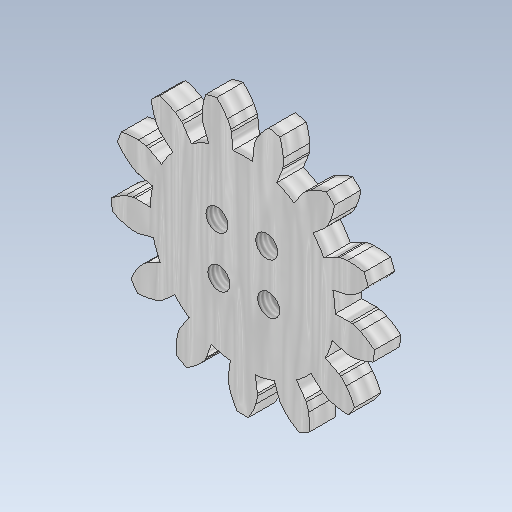
# Autodesk Inventor part: ｍ2歯数13ギアd10同軸ネジ切甲
Saved by Autodesk Inventor 2020.2 (Build 242310000, 310)
## iProperties
Created: 2020-02-11
Part Number: ｍ2歯数13ギアd10同軸ネジ切甲
Material: アルミニウム 7075
Document SubType Name: Modeling
Designer: aoyam
Density: 2.81 g/cm^3
Appearance: サテン - ブラシ仕上げ 重厚
Author: aoyam
Autodesk Inventor part; units mm, degrees
ref_plane "YZ Plane" through (0, 0, 0) normal (1, 0, 0) x (0, 1, 0)
ref_plane "XZ Plane" through (0, 0, 0) normal (0, 1, 0) x (-1, 0, 0)
ref_plane "XY Plane" through (0, 0, 0) normal (0, 0, 1) x (1, 0, 0)
sketch "スケッチ1" plane through (0, 0, 0) normal (0, 0, 1) x (1, 0, 0)
  arc A0 (149.8566, 117.4069) -> (149.7916, 117.1475) centre (151.2088, 116.9303) ccw
  arc A1 (150.243, 118.2214) -> (149.8566, 117.4069) centre (153.6231, 116.1188) ccw
  arc A2 (151.4709, 119.7028) -> (150.243, 118.2214) centre (156.2171, 114.5193) ccw
  arc A3 (147.2084, 117.1475) -> (147.1434, 117.4069) centre (145.7912, 116.9303) ccw
  arc A4 (147.1434, 117.4069) -> (146.757, 118.2214) centre (143.3769, 116.1188) ccw
  arc A5 (146.757, 118.2214) -> (145.5291, 119.7028) centre (140.7829, 114.5193) ccw
  arc A6 (149.6101, 115.4411) -> (147.3899, 115.4411) centre (148.5, 105) ccw
  arc A7 (145.5291, 119.7028) -> (144.2978, 119.3994) centre (148.5, 105) ccw
  line L0 (149.6101, 115.4411) -> (149.7916, 117.1475)
  line L1 (147.3899, 115.4411) -> (147.2084, 117.1475)
  line L2 (131.5, 105) -> (165.5, 105)
  line L3 (148.5, 88) -> (148.5, 122)
  arc A8 (143.9354, 116.6162) -> (143.9984, 116.3563) centre (145.3542, 116.8225) ccw
  line L4 (144.6307, 114.7611) -> (143.9984, 116.3563)
  arc A9 (143.8991, 117.517) -> (143.9354, 116.6162) centre (147.8691, 117.226) ccw
  arc A10 (144.2978, 119.3994) -> (143.8991, 117.517) centre (150.9093, 117.0153) ccw
  arc A11 (144.6307, 114.7611) -> (142.6648, 113.7293) centre (148.5, 105) ccw
  line L5 (142.6648, 113.7293) -> (141.7111, 115.1559)
  arc A12 (141.7111, 115.1559) -> (141.5331, 115.3553) centre (140.5572, 114.3049) ccw
  arc A13 (141.5331, 115.3553) -> (140.8123, 115.897) centre (138.7966, 112.4644) ccw
  arc A14 (140.8123, 115.897) -> (139.0366, 116.6381) centre (137.2429, 109.8426) ccw
  arc A15 (139.0366, 116.6381) -> (138.0875, 115.7972) centre (148.5, 105) ccw
  arc A16 (139.0599, 113.1643) -> (139.2365, 112.9635) centre (140.2203, 114.0064) ccw
  line L6 (140.5377, 111.8449) -> (139.2365, 112.9635)
  arc A17 (138.6091, 113.9451) -> (139.0599, 113.1643) centre (142.2596, 115.5324) ccw
  arc A18 (138.0875, 115.7972) -> (138.6091, 113.9451) centre (145.0496, 116.7587) ccw
  arc A19 (140.5377, 111.8449) -> (139.2765, 110.0176) centre (148.5, 105) ccw
  line L7 (139.2765, 110.0176) -> (137.7691, 110.8376)
  arc A20 (137.7691, 110.8376) -> (137.5187, 110.9315) centre (137.1428, 109.5479) ccw
  arc A21 (137.5187, 110.9315) -> (136.6288, 111.0762) centre (136.4392, 107.1) ccw
  arc A22 (136.6288, 111.0762) -> (134.7121, 110.9072) centre (136.2819, 104.0565) ccw
  arc A23 (134.7121, 110.9072) -> (134.2625, 109.7215) centre (148.5, 105) ccw
  arc A24 (136.3471, 107.8422) -> (136.5967, 107.7464) centre (136.9832, 109.127) ccw
  line L8 (138.2688, 107.3606) -> (136.5967, 107.7464)
  arc A25 (135.585, 108.324) -> (136.3471, 107.8422) centre (138.0798, 111.426) ccw
  arc A26 (134.2625, 109.7215) -> (135.585, 108.324) centre (139.9803, 113.8083) ccw
  arc A27 (138.2688, 107.3606) -> (138.0012, 105.1565) centre (148.5, 105) ccw
  line L9 (138.0012, 105.1565) -> (136.2854, 105.1821)
  arc A28 (136.2854, 105.1821) -> (136.0201, 105.1488) centre (136.3302, 103.749) ccw
  arc A29 (136.0201, 105.1488) -> (135.1649, 104.8633) centre (136.8447, 101.2545) ccw
  arc A30 (135.1649, 104.8633) -> (133.5462, 103.823) centre (138.1199, 98.4866) ccw
  arc A31 (133.5462, 103.823) -> (133.6991, 102.5641) centre (148.5, 105) ccw
  arc A32 (136.4183, 101.8689) -> (136.6839, 101.9001) centre (136.3845, 103.3022) ccw
  line L10 (138.3437, 102.3355) -> (136.6839, 101.9001)
  arc A33 (135.5196, 101.9414) -> (136.4183, 101.8689) centre (136.2871, 105.8474) ccw
  arc A34 (133.6991, 102.5641) -> (135.5196, 101.9414) centre (136.8627, 108.84) ccw
  arc A35 (138.3437, 102.3355) -> (139.131, 100.2595) centre (148.5, 105) ccw
  line L11 (139.131, 100.2595) -> (137.5999, 99.4848)
  arc A36 (137.5999, 99.4848) -> (137.3804, 99.3321) centre (138.3055, 98.2367) ccw
  arc A37 (137.3804, 99.3321) -> (136.7558, 98.6818) centre (139.9204, 96.2671) ccw
  arc A38 (136.7558, 98.6818) -> (135.8061, 97.0085) centre (142.3358, 94.4087) ccw
  arc A39 (135.8061, 97.0085) -> (136.5265, 95.9648) centre (148.5, 105) ccw
  arc A40 (139.2573, 96.6129) -> (139.4779, 96.7639) centre (138.5612, 97.8663) ccw
  line L12 (140.7453, 97.9209) -> (139.4779, 96.7639)
  arc A41 (138.4279, 96.2594) -> (139.2573, 96.6129) centre (137.2922, 100.0747) ccw
  arc A42 (136.5265, 95.9648) -> (138.4279, 96.2594) centre (136.4111, 102.9921) ccw
  arc A43 (140.7453, 97.9209) -> (142.4072, 96.4485) centre (148.5, 105) ccw
  line L13 (142.4072, 96.4485) -> (141.4115, 95.051)
  arc A44 (141.4115, 95.051) -> (141.2881, 94.8138) centre (142.6163, 94.2738) ccw
  arc A45 (141.2881, 94.8138) -> (141.0372, 93.9478) centre (144.9616, 93.2802) ccw
  arc A46 (141.0372, 93.9478) -> (140.974, 92.0247) centre (147.9639, 92.7573) ccw
  arc A47 (140.974, 92.0247) -> (142.0968, 91.4354) centre (148.5, 105) ccw
  arc A48 (144.2137, 93.2783) -> (144.3389, 93.5145) centre (143.0149, 94.0647) ccw
  line L14 (144.9234, 95.1279) -> (144.3389, 93.5145)
  arc A49 (143.6435, 92.5799) -> (144.2137, 93.2783) centre (140.8649, 95.4303) ccw
  arc A50 (142.0968, 91.4354) -> (143.6435, 92.5799) centre (138.729, 97.6041) ccw
  arc A51 (144.9234, 95.1279) -> (147.0792, 94.5966) centre (148.5, 105) ccw
  line L15 (147.0792, 94.5966) -> (146.8469, 92.8964)
  arc A52 (146.8469, 92.8964) -> (146.848, 92.629) centre (148.2749, 92.7682) ccw
  arc A53 (146.848, 92.629) -> (147.0283, 91.7456) centre (150.8133, 92.9783) ccw
  arc A54 (147.0283, 91.7456) -> (147.8659, 90.0134) centre (153.7148, 93.9104) ccw
  arc A55 (147.8659, 90.0134) -> (149.1341, 90.0134) centre (148.5, 105) ccw
  arc A56 (150.152, 92.629) -> (150.1531, 92.8964) centre (148.7251, 92.7682) ccw
  line L16 (149.9208, 94.5966) -> (150.1531, 92.8964)
  arc A57 (149.9717, 91.7456) -> (150.152, 92.629) centre (146.1867, 92.9783) ccw
  arc A58 (149.1341, 90.0134) -> (149.9717, 91.7456) centre (143.2852, 93.9104) ccw
  arc A59 (149.9208, 94.5966) -> (152.0766, 95.1279) centre (148.5, 105) ccw
  line L17 (152.0766, 95.1279) -> (152.6611, 93.5145)
  arc A60 (152.6611, 93.5145) -> (152.7863, 93.2783) centre (153.9851, 94.0647) ccw
  arc A61 (152.7863, 93.2783) -> (153.3565, 92.5799) centre (156.1351, 95.4303) ccw
  arc A62 (153.3565, 92.5799) -> (154.9032, 91.4354) centre (158.271, 97.6041) ccw
  arc A63 (154.9032, 91.4354) -> (156.026, 92.0247) centre (148.5, 105) ccw
  arc A64 (155.7119, 94.8138) -> (155.5885, 95.051) centre (154.3837, 94.2738) ccw
  line L18 (154.5928, 96.4485) -> (155.5885, 95.051)
  arc A65 (155.9628, 93.9478) -> (155.7119, 94.8138) centre (152.0384, 93.2802) ccw
  arc A66 (156.026, 92.0247) -> (155.9628, 93.9478) centre (149.0361, 92.7573) ccw
  arc A67 (154.5928, 96.4485) -> (156.2547, 97.9209) centre (148.5, 105) ccw
  line L19 (156.2547, 97.9209) -> (157.5221, 96.7639)
  arc A68 (157.5221, 96.7639) -> (157.7427, 96.6129) centre (158.4388, 97.8663) ccw
  arc A69 (157.7427, 96.6129) -> (158.5721, 96.2594) centre (159.7078, 100.0747) ccw
  arc A70 (158.5721, 96.2594) -> (160.4735, 95.9648) centre (160.5889, 102.9921) ccw
  arc A71 (160.4735, 95.9648) -> (161.1939, 97.0085) centre (148.5, 105) ccw
  arc A72 (159.6196, 99.3321) -> (159.4001, 99.4848) centre (158.6945, 98.2367) ccw
  line L20 (157.869, 100.2595) -> (159.4001, 99.4848)
  arc A73 (160.2442, 98.6818) -> (159.6196, 99.3321) centre (157.0796, 96.2671) ccw
  arc A74 (161.1939, 97.0085) -> (160.2442, 98.6818) centre (154.6642, 94.4087) ccw
  arc A75 (157.869, 100.2595) -> (158.6563, 102.3355) centre (148.5, 105) ccw
  line L21 (158.6563, 102.3355) -> (160.3161, 101.9001)
  arc A76 (160.3161, 101.9001) -> (160.5817, 101.8689) centre (160.6155, 103.3022) ccw
  arc A77 (160.5817, 101.8689) -> (161.4804, 101.9414) centre (160.7129, 105.8474) ccw
  arc A78 (161.4804, 101.9414) -> (163.3009, 102.5641) centre (160.1373, 108.84) ccw
  arc A79 (163.3009, 102.5641) -> (163.4538, 103.823) centre (148.5, 105) ccw
  arc A80 (160.9799, 105.1488) -> (160.7146, 105.1821) centre (160.6698, 103.749) ccw
  line L22 (158.9988, 105.1565) -> (160.7146, 105.1821)
  arc A81 (161.8351, 104.8633) -> (160.9799, 105.1488) centre (160.1553, 101.2545) ccw
  arc A82 (163.4538, 103.823) -> (161.8351, 104.8633) centre (158.8801, 98.4866) ccw
  arc A83 (158.9988, 105.1565) -> (158.7312, 107.3606) centre (148.5, 105) ccw
  line L23 (158.7312, 107.3606) -> (160.4033, 107.7464)
  arc A84 (160.4033, 107.7464) -> (160.6529, 107.8422) centre (160.0168, 109.127) ccw
  arc A85 (160.6529, 107.8422) -> (161.415, 108.324) centre (158.9202, 111.426) ccw
  arc A86 (161.415, 108.324) -> (162.7375, 109.7215) centre (157.0197, 113.8083) ccw
  arc A87 (162.7375, 109.7215) -> (162.2879, 110.9072) centre (148.5, 105) ccw
  arc A88 (159.4813, 110.9315) -> (159.2309, 110.8376) centre (159.8572, 109.5479) ccw
  line L24 (157.7235, 110.0176) -> (159.2309, 110.8376)
  arc A89 (160.3712, 111.0762) -> (159.4813, 110.9315) centre (160.5608, 107.1) ccw
  arc A90 (162.2879, 110.9072) -> (160.3712, 111.0762) centre (160.7181, 104.0565) ccw
  arc A91 (157.7235, 110.0176) -> (156.4623, 111.8449) centre (148.5, 105) ccw
  line L25 (156.4623, 111.8449) -> (157.7635, 112.9635)
  arc A92 (157.7635, 112.9635) -> (157.9401, 113.1643) centre (156.7797, 114.0064) ccw
  arc A93 (157.9401, 113.1643) -> (158.3909, 113.9451) centre (154.7404, 115.5324) ccw
  arc A94 (158.3909, 113.9451) -> (158.9125, 115.7972) centre (151.9504, 116.7587) ccw
  arc A95 (158.9125, 115.7972) -> (157.9634, 116.6381) centre (148.5, 105) ccw
  arc A96 (155.4669, 115.3553) -> (155.2889, 115.1559) centre (156.4428, 114.3049) ccw
  line L26 (154.3352, 113.7293) -> (155.2889, 115.1559)
  arc A97 (156.1877, 115.897) -> (155.4669, 115.3553) centre (158.2034, 112.4644) ccw
  arc A98 (157.9634, 116.6381) -> (156.1877, 115.897) centre (159.7571, 109.8426) ccw
  arc A99 (154.3352, 113.7293) -> (152.3693, 114.7611) centre (148.5, 105) ccw
  line L27 (152.3693, 114.7611) -> (153.0016, 116.3563)
  arc A100 (153.0016, 116.3563) -> (153.0646, 116.6162) centre (151.6458, 116.8225) ccw
  arc A101 (153.0646, 116.6162) -> (153.1009, 117.517) centre (149.1309, 117.226) ccw
  arc A102 (153.1009, 117.517) -> (152.7022, 119.3994) centre (146.0907, 117.0153) ccw
  arc A103 (152.7022, 119.3994) -> (151.4709, 119.7028) centre (148.5, 105) ccw
  circle A104 centre (148.5, 105) radius 10.5
  circle A105 centre (148.5, 105) radius 7.75 construction
  circle A106 centre (145.5628, 107.7153) radius 1.25
  circle A107 centre (145.7847, 102.0628) radius 1.25
  circle A108 centre (151.4372, 102.2847) radius 1.25
  circle A109 centre (151.2153, 107.9372) radius 1.25
  line L28 (142.8007, 109.2819) -> (145.5384, 110.8906)
  line L29 (145.5384, 110.8906) -> (148.3005, 109.324)
  line L30 (148.3005, 109.324) -> (148.3249, 106.1487)
  line L31 (148.3249, 106.1487) -> (145.5871, 104.5399)
  line L32 (145.5871, 104.5399) -> (142.825, 106.1065)
  line L33 (142.825, 106.1065) -> (142.8007, 109.2819)
  circle A110 centre (145.5628, 107.7153) radius 3.1754
  circle A111 centre (151.2153, 107.9372) radius 2.75
  point P0 (0, 0)
  point P1 (140.5997, 120.0528)
  point P2 (134.5093, 114.6571)
  point P3 (131.6239, 107.0491)
  point P4 (132.6047, 98.9717)
  point P5 (137.2269, 92.2753)
  point P6 (144.4316, 88.494)
  point P7 (152.5684, 88.494)
  point P8 (159.7731, 92.2753)
  point P9 (164.3953, 98.9717)
  point P10 (165.3761, 107.0491)
  point P11 (162.4907, 114.6571)
  point P12 (156.4003, 120.0528)
  point P13 (149.1341, 90.0134)
  point P14 (149.9717, 91.7456)
  point P15 (150.152, 92.629)
  point P16 (149.9208, 94.5966)
  point P17 (152.7863, 93.2783)
  point P18 (153.3565, 92.5799)
  point P19 (154.9032, 91.4354)
  point P20 (156.026, 92.0247)
  point P21 (155.9628, 93.9478)
  point P22 (154.5928, 96.4485)
  point P23 (157.5221, 96.7639)
  point P24 (157.7427, 96.6129)
  point P25 (158.5721, 96.2594)
  point P26 (160.4735, 95.9648)
  point P27 (161.1939, 97.0085)
  point P28 (160.2442, 98.6818)
  point P29 (160.3161, 101.9001)
  point P30 (160.5817, 101.8689)
  point P31 (161.4804, 101.9414)
  point P32 (161.8351, 104.8633)
  point P33 (160.6529, 107.8422)
  point P34 (162.7375, 109.7215)
  point P35 (162.2879, 110.9072)
  point P36 (160.3712, 111.0762)
  point P37 (159.4813, 110.9315)
  point P38 (157.7235, 110.0176)
  point P39 (157.7635, 112.9635)
  point P40 (157.9401, 113.1643)
  point P41 (158.3909, 113.9451)
  point P42 (158.9125, 115.7972)
  point P43 (154.3352, 113.7293)
  point P44 (153.0016, 116.3563)
  point P45 (152.7022, 119.3994)
  point P46 (151.4709, 119.7028)
  point P47 (150.243, 118.2214)
  point P48 (149.8566, 117.4069)
  point P49 (147.3899, 115.4411)
  point P50 (146.757, 118.2214)
  point P51 (144.2978, 119.3994)
  point P52 (143.8991, 117.517)
  point P53 (144.6307, 114.7611)
  point P54 (140.8123, 115.897)
  point P55 (139.0366, 116.6381)
  point P56 (138.0875, 115.7972)
  point P57 (138.6091, 113.9451)
  point P58 (139.0599, 113.1643)
  point P59 (140.5377, 111.8449)
  point P60 (137.7691, 110.8376)
  point P61 (137.5187, 110.9315)
  point P62 (136.6288, 111.0762)
  point P63 (134.7121, 110.9072)
  point P64 (134.2625, 109.7215)
  point P65 (135.585, 108.324)
  point P66 (138.2688, 107.3606)
  point P67 (133.5462, 103.823)
  point P68 (133.6991, 102.5641)
  point P69 (135.5196, 101.9414)
  point P70 (136.4183, 101.8689)
  point P71 (138.3437, 102.3355)
  point P72 (137.5999, 99.4848)
  point P73 (137.3804, 99.3321)
  point P74 (142.0968, 91.4354)
  point P75 (144.2137, 93.2783)
  point P76 (147.8659, 90.0134)
  dimension "d25" = 6.3509
  dimension "d2" = 360
  dimension "d16" = 2.5
  dimension "d17" = 4
  dimension "d20" = 360
  dimension "d24" = 5.5
  dimension "d26" = 5.5
  constraints: 208 point on circle, 111 centre point, 68 end point, 6 coincident, 1 concentric, 1 midpoint, 532 other
  measures "d16" diameter of A106
  measures "d17" distance of A6.centre A106.centre
  measures "d24" distance between parallel lines of L32 L29
  measures "d26" diameter of A111
extrude "押し出し1" add sketch "スケッチ1" along normal blind 3
sketch "スケッチ2" plane through (0, 0, 0) normal (0, 0, -1) x (-1, 0, 0)
  point P0 (0, 0)
sketch "スケッチ3" plane through (0, 0, 3) normal (0, 0, 1) x (1, 0, 0)
  arc A0 (138.4279, 96.2594) -> (139.2573, 96.6129) centre (137.2922, 100.0747) ccw projected
  arc A1 (139.2573, 96.6129) -> (139.4779, 96.7639) centre (138.5612, 97.8663) ccw projected
  line L0 (139.4779, 96.7639) -> (140.7453, 97.9209) projected
  arc A2 (140.7453, 97.9209) -> (142.4072, 96.4485) centre (148.5, 105) ccw projected
  line L1 (142.4072, 96.4485) -> (141.4115, 95.051) projected
  arc A3 (141.4115, 95.051) -> (141.2881, 94.8138) centre (142.6163, 94.2738) ccw projected
  arc A4 (141.2881, 94.8138) -> (141.0372, 93.9478) centre (144.9616, 93.2802) ccw projected
  arc A5 (141.0372, 93.9478) -> (140.974, 92.0247) centre (147.9639, 92.7573) ccw projected
  arc A6 (140.974, 92.0247) -> (142.0968, 91.4354) centre (148.5, 105) ccw projected
  arc A7 (142.0968, 91.4354) -> (143.6435, 92.5799) centre (138.729, 97.6041) ccw projected
  arc A8 (143.6435, 92.5799) -> (144.2137, 93.2783) centre (140.8649, 95.4303) ccw projected
  arc A9 (144.2137, 93.2783) -> (144.3389, 93.5145) centre (143.0149, 94.0647) ccw projected
  line L2 (144.3389, 93.5145) -> (144.9234, 95.1279) projected
  arc A10 (144.9234, 95.1279) -> (147.0792, 94.5966) centre (148.5, 105) ccw projected
  line L3 (147.0792, 94.5966) -> (146.8469, 92.8964) projected
  arc A11 (146.8469, 92.8964) -> (146.848, 92.629) centre (148.2749, 92.7682) ccw projected
  arc A12 (146.848, 92.629) -> (147.0283, 91.7456) centre (150.8133, 92.9783) ccw projected
  arc A13 (147.0283, 91.7456) -> (147.8659, 90.0134) centre (153.7148, 93.9104) ccw projected
  arc A14 (147.8659, 90.0134) -> (149.1341, 90.0134) centre (148.5, 105) ccw projected
  arc A15 (149.1341, 90.0134) -> (149.9717, 91.7456) centre (143.2852, 93.9104) ccw projected
  arc A16 (149.9717, 91.7456) -> (150.152, 92.629) centre (146.1867, 92.9783) ccw projected
  arc A17 (150.152, 92.629) -> (150.1531, 92.8964) centre (148.7251, 92.7682) ccw projected
  line L4 (150.1531, 92.8964) -> (149.9208, 94.5966) projected
  arc A18 (149.9208, 94.5966) -> (152.0766, 95.1279) centre (148.5, 105) ccw projected
  line L5 (152.0766, 95.1279) -> (152.6611, 93.5145) projected
  arc A19 (152.6611, 93.5145) -> (152.7863, 93.2783) centre (153.9851, 94.0647) ccw projected
  arc A20 (152.7863, 93.2783) -> (153.3565, 92.5799) centre (156.1351, 95.4303) ccw projected
  arc A21 (153.3565, 92.5799) -> (154.9032, 91.4354) centre (158.271, 97.6041) ccw projected
  arc A22 (154.9032, 91.4354) -> (156.026, 92.0247) centre (148.5, 105) ccw projected
  arc A23 (156.026, 92.0247) -> (155.9628, 93.9478) centre (149.0361, 92.7573) ccw projected
  arc A24 (155.9628, 93.9478) -> (155.7119, 94.8138) centre (152.0384, 93.2802) ccw projected
  arc A25 (155.7119, 94.8138) -> (155.5885, 95.051) centre (154.3837, 94.2738) ccw projected
  line L6 (155.5885, 95.051) -> (154.5928, 96.4485) projected
  arc A26 (154.5928, 96.4485) -> (156.2547, 97.9209) centre (148.5, 105) ccw projected
  line L7 (156.2547, 97.9209) -> (157.5221, 96.7639) projected
  arc A27 (157.5221, 96.7639) -> (157.7427, 96.6129) centre (158.4388, 97.8663) ccw projected
  arc A28 (157.7427, 96.6129) -> (158.5721, 96.2594) centre (159.7078, 100.0747) ccw projected
  arc A29 (158.5721, 96.2594) -> (160.4735, 95.9648) centre (160.5889, 102.9921) ccw projected
  arc A30 (160.4735, 95.9648) -> (161.1939, 97.0085) centre (148.5, 105) ccw projected
  arc A31 (161.1939, 97.0085) -> (160.2442, 98.6818) centre (154.6642, 94.4087) ccw projected
  arc A32 (160.2442, 98.6818) -> (159.6196, 99.3321) centre (157.0796, 96.2671) ccw projected
  arc A33 (159.6196, 99.3321) -> (159.4001, 99.4848) centre (158.6945, 98.2367) ccw projected
  line L8 (159.4001, 99.4848) -> (157.869, 100.2595) projected
  arc A34 (157.869, 100.2595) -> (158.6563, 102.3355) centre (148.5, 105) ccw projected
  line L9 (158.6563, 102.3355) -> (160.3161, 101.9001) projected
  arc A35 (160.3161, 101.9001) -> (160.5817, 101.8689) centre (160.6155, 103.3022) ccw projected
  arc A36 (160.5817, 101.8689) -> (161.4804, 101.9414) centre (160.7129, 105.8474) ccw projected
  arc A37 (161.4804, 101.9414) -> (163.3009, 102.5641) centre (160.1373, 108.84) ccw projected
  arc A38 (163.3009, 102.5641) -> (163.4538, 103.823) centre (148.5, 105) ccw projected
  arc A39 (163.4538, 103.823) -> (161.8351, 104.8633) centre (158.8801, 98.4866) ccw projected
  arc A40 (161.8351, 104.8633) -> (160.9799, 105.1488) centre (160.1553, 101.2545) ccw projected
  arc A41 (160.9799, 105.1488) -> (160.7146, 105.1821) centre (160.6698, 103.749) ccw projected
  line L10 (160.7146, 105.1821) -> (158.9988, 105.1565) projected
  arc A42 (158.9988, 105.1565) -> (158.7312, 107.3606) centre (148.5, 105) ccw projected
  line L11 (158.7312, 107.3606) -> (160.4033, 107.7464) projected
  arc A43 (160.4033, 107.7464) -> (160.6529, 107.8422) centre (160.0168, 109.127) ccw projected
  arc A44 (160.6529, 107.8422) -> (161.415, 108.324) centre (158.9202, 111.426) ccw projected
  arc A45 (161.415, 108.324) -> (162.7375, 109.7215) centre (157.0197, 113.8083) ccw projected
  arc A46 (162.7375, 109.7215) -> (162.2879, 110.9072) centre (148.5, 105) ccw projected
  arc A47 (162.2879, 110.9072) -> (160.3712, 111.0762) centre (160.7181, 104.0565) ccw projected
  arc A48 (160.3712, 111.0762) -> (159.4813, 110.9315) centre (160.5608, 107.1) ccw projected
  arc A49 (159.4813, 110.9315) -> (159.2309, 110.8376) centre (159.8572, 109.5479) ccw projected
  line L12 (159.2309, 110.8376) -> (157.7235, 110.0176) projected
  arc A50 (157.7235, 110.0176) -> (156.4623, 111.8449) centre (148.5, 105) ccw projected
  line L13 (156.4623, 111.8449) -> (157.7635, 112.9635) projected
  arc A51 (157.7635, 112.9635) -> (157.9401, 113.1643) centre (156.7797, 114.0064) ccw projected
  arc A52 (157.9401, 113.1643) -> (158.3909, 113.9451) centre (154.7404, 115.5324) ccw projected
  arc A53 (158.3909, 113.9451) -> (158.9125, 115.7972) centre (151.9504, 116.7587) ccw projected
  arc A54 (158.9125, 115.7972) -> (157.9634, 116.6381) centre (148.5, 105) ccw projected
  arc A55 (157.9634, 116.6381) -> (156.1877, 115.897) centre (159.7571, 109.8426) ccw projected
  arc A56 (156.1877, 115.897) -> (155.4669, 115.3553) centre (158.2034, 112.4644) ccw projected
  arc A57 (155.4669, 115.3553) -> (155.2889, 115.1559) centre (156.4428, 114.3049) ccw projected
  line L14 (155.2889, 115.1559) -> (154.3352, 113.7293) projected
  arc A58 (154.3352, 113.7293) -> (152.3693, 114.7611) centre (148.5, 105) ccw projected
  line L15 (152.3693, 114.7611) -> (153.0016, 116.3563) projected
  arc A59 (153.0016, 116.3563) -> (153.0646, 116.6162) centre (151.6458, 116.8225) ccw projected
  arc A60 (153.0646, 116.6162) -> (153.1009, 117.517) centre (149.1309, 117.226) ccw projected
  arc A61 (153.1009, 117.517) -> (152.7022, 119.3994) centre (146.0907, 117.0153) ccw projected
  arc A62 (152.7022, 119.3994) -> (151.4709, 119.7028) centre (148.5, 105) ccw projected
  arc A63 (151.4709, 119.7028) -> (150.243, 118.2214) centre (156.2171, 114.5193) ccw projected
  arc A64 (150.243, 118.2214) -> (149.8566, 117.4069) centre (153.6231, 116.1188) ccw projected
  arc A65 (149.8566, 117.4069) -> (149.7916, 117.1475) centre (151.2088, 116.9303) ccw projected
  line L16 (149.7916, 117.1475) -> (149.6101, 115.4411) projected
  arc A66 (149.6101, 115.4411) -> (147.3899, 115.4411) centre (148.5, 105) ccw projected
  line L17 (147.3899, 115.4411) -> (147.2084, 117.1475) projected
  arc A67 (147.2084, 117.1475) -> (147.1434, 117.4069) centre (145.7912, 116.9303) ccw projected
  arc A68 (147.1434, 117.4069) -> (146.757, 118.2214) centre (143.3769, 116.1188) ccw projected
  arc A69 (146.757, 118.2214) -> (145.5291, 119.7028) centre (140.7829, 114.5193) ccw projected
  arc A70 (145.5291, 119.7028) -> (144.2978, 119.3994) centre (148.5, 105) ccw projected
  arc A71 (144.2978, 119.3994) -> (143.8991, 117.517) centre (150.9093, 117.0153) ccw projected
  arc A72 (143.8991, 117.517) -> (143.9354, 116.6162) centre (147.8691, 117.226) ccw projected
  arc A73 (143.9354, 116.6162) -> (143.9984, 116.3563) centre (145.3542, 116.8225) ccw projected
  line L18 (143.9984, 116.3563) -> (144.6307, 114.7611) projected
  arc A74 (144.6307, 114.7611) -> (142.6648, 113.7293) centre (148.5, 105) ccw projected
  line L19 (142.6648, 113.7293) -> (141.7111, 115.1559) projected
  arc A75 (141.7111, 115.1559) -> (141.5331, 115.3553) centre (140.5572, 114.3049) ccw projected
  arc A76 (141.5331, 115.3553) -> (140.8123, 115.897) centre (138.7966, 112.4644) ccw projected
  arc A77 (140.8123, 115.897) -> (139.0366, 116.6381) centre (137.2429, 109.8426) ccw projected
  arc A78 (139.0366, 116.6381) -> (138.0875, 115.7972) centre (148.5, 105) ccw projected
  arc A79 (138.0875, 115.7972) -> (138.6091, 113.9451) centre (145.0496, 116.7587) ccw projected
  arc A80 (138.6091, 113.9451) -> (139.0599, 113.1643) centre (142.2596, 115.5324) ccw projected
  arc A81 (139.0599, 113.1643) -> (139.2365, 112.9635) centre (140.2203, 114.0064) ccw projected
  line L20 (139.2365, 112.9635) -> (140.5377, 111.8449) projected
  arc A82 (140.5377, 111.8449) -> (139.2765, 110.0176) centre (148.5, 105) ccw projected
  line L21 (139.2765, 110.0176) -> (137.7691, 110.8376) projected
  arc A83 (137.7691, 110.8376) -> (137.5187, 110.9315) centre (137.1428, 109.5479) ccw projected
  arc A84 (137.5187, 110.9315) -> (136.6288, 111.0762) centre (136.4392, 107.1) ccw projected
  arc A85 (136.6288, 111.0762) -> (134.7121, 110.9072) centre (136.2819, 104.0565) ccw projected
  arc A86 (134.7121, 110.9072) -> (134.2625, 109.7215) centre (148.5, 105) ccw projected
  arc A87 (134.2625, 109.7215) -> (135.585, 108.324) centre (139.9803, 113.8083) ccw projected
  arc A88 (135.585, 108.324) -> (136.3471, 107.8422) centre (138.0798, 111.426) ccw projected
  arc A89 (136.3471, 107.8422) -> (136.5967, 107.7464) centre (136.9832, 109.127) ccw projected
  line L22 (136.5967, 107.7464) -> (138.2688, 107.3606) projected
  arc A90 (138.2688, 107.3606) -> (138.0012, 105.1565) centre (148.5, 105) ccw projected
  line L23 (138.0012, 105.1565) -> (136.2854, 105.1821) projected
  arc A91 (136.2854, 105.1821) -> (136.0201, 105.1488) centre (136.3302, 103.749) ccw projected
  arc A92 (136.0201, 105.1488) -> (135.1649, 104.8633) centre (136.8447, 101.2545) ccw projected
  arc A93 (135.1649, 104.8633) -> (133.5462, 103.823) centre (138.1199, 98.4866) ccw projected
  arc A94 (133.5462, 103.823) -> (133.6991, 102.5641) centre (148.5, 105) ccw projected
  arc A95 (133.6991, 102.5641) -> (135.5196, 101.9414) centre (136.8627, 108.84) ccw projected
  arc A96 (135.5196, 101.9414) -> (136.4183, 101.8689) centre (136.2871, 105.8474) ccw projected
  arc A97 (136.4183, 101.8689) -> (136.6839, 101.9001) centre (136.3845, 103.3022) ccw projected
  line L24 (136.6839, 101.9001) -> (138.3437, 102.3355) projected
  arc A98 (138.3437, 102.3355) -> (139.131, 100.2595) centre (148.5, 105) ccw projected
  line L25 (139.131, 100.2595) -> (137.5999, 99.4848) projected
  arc A99 (137.5999, 99.4848) -> (137.3804, 99.3321) centre (138.3055, 98.2367) ccw projected
  arc A100 (137.3804, 99.3321) -> (136.7558, 98.6818) centre (139.9204, 96.2671) ccw projected
  arc A101 (136.7558, 98.6818) -> (135.8061, 97.0085) centre (142.3358, 94.4087) ccw projected
  arc A102 (135.8061, 97.0085) -> (136.5265, 95.9648) centre (148.5, 105) ccw projected
  arc A103 (136.5265, 95.9648) -> (138.4279, 96.2594) centre (136.4111, 102.9921) ccw projected
  circle A104 centre (145.5628, 107.7153) radius 1.25 projected
  circle A105 centre (151.4372, 102.2847) radius 1.25 projected
  circle A106 centre (151.2153, 107.9372) radius 1.25 projected
  circle A107 centre (145.7847, 102.0628) radius 1.25 projected
  circle A108 centre (148.5, 105) radius 2.75
  circle A109 centre (148.5, 105) radius 5.75
  point P0 (0, 0)
  dimension "d22" = 3
  dimension "d23" = 11.5
  constraints: 2 centre point, 1 coincident, 1 tangent
  measures "d22" radial gap between concentric circles of A108 A109
  measures "d23" diameter of A109
sketch "スケッチ4" plane through (0, 0, 3) normal (0, 0, 1) x (1, 0, 0)
  circle A0 centre (145.5628, 107.7153) radius 1.25 projected
  circle A1 centre (151.2153, 107.9372) radius 1.25 projected
  circle A2 centre (145.7847, 102.0628) radius 1.25 projected
  circle A3 centre (151.4372, 102.2847) radius 1.25 projected
  arc A4 (149.6101, 115.4411) -> (147.3899, 115.4411) centre (148.5, 105) ccw projected
  point P0 (0, 0)
thread "ねじ1" size "M3x0.5" class "6H" standard "ANSI Metric M Profile" length 100
thread "ねじ2" size "M3x0.5" class "6H" standard "ANSI Metric M Profile" length 100
thread "ねじ3" size "M3x0.5" class "6H" standard "ANSI Metric M Profile" length 100
thread "ねじ4" size "M3x0.5" class "6H" standard "ANSI Metric M Profile" length 100
